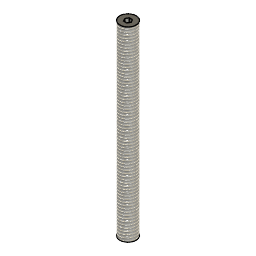
DoubleBarrelHotend (Autodesk Fusion 360 archive; units mm, degrees)
design "meltzone adapter"
Autodesk Fusion 360 part; units mm, degrees
sketch "Sketch1" plane through (0, 0, 0) normal (0, 0, 1) x (1, 0, 0)
  circle A0 centre (0, 0) radius 3
  circle A1 centre (0, 0) radius 1
  dimension "d1" = 6
  dimension "d2" = 2
  constraint coincident A0.centre A1.centre
  measures "d1" diameter of A0
  measures "d2" diameter of A1
extrude "Extrude1" add sketch "Sketch1" along normal blind 67
thread "Thread1" "ISO Metric profile 6.0 M6x1 M6x1 6g" major diameter 5.884 minor diameter 4.7435 pitch 1 angle 60 resizes the face on face at (2.9963, -0.1495, 44.6667)
sketch "Sketch2" plane through (0, 0, 67) normal (0, 0, 1) x (-1, 0, 0)
  circle A0 centre (0, 0) radius 1
  circle A1 centre (0, 0) radius 2.942
  line L0 (0.5774, -1) -> (1.1547, 0)
  line L1 (1.1547, 0) -> (0.5774, 1)
  line L2 (0.5774, 1) -> (-0.5774, 1)
  line L3 (-0.5774, 1) -> (-1.1547, 0)
  line L4 (-1.1547, 0) -> (-0.5774, -1)
  line L5 (-0.5774, -1) -> (0.5774, -1)
  constraint coincident A0.centre A1.centre
extrude "Extrude2" cut sketch "Sketch2" against normal blind 2 contours A0 | A0 L0 L1 | A0 L1 L2 | A0 L0 L5 | A0 L2 L3 | A0 L4 L5 | A0 L3 L4

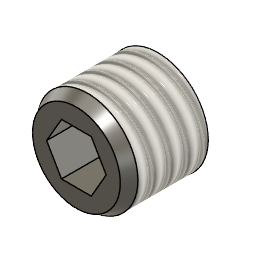
design "Hexagon Socket Set Screw ISO 4027 - M3 x 3 Steel 4.6 Plain"
description: Hexagon Socket Set Screw ISO 4027 - M3 x 3
part number: ISO 4027 - M3 x 3 Steel 4.6 Plain
Autodesk Fusion 360 part; units mm, degrees
sketch "Sketch1" plane through (0, 0, 0) normal (0, 1, 0) x (1, 0, 0)
  line L0 (-1.5, 0) -> (-1.5, 3)
  line L1 (0, 3) -> (0, 0)
  line L2 (0, 3) -> (-1.5, 3)
  line L3 (-1.5, 0) -> (0, 0)
  dimension "d107" = 3
  dimension "d136" = 3
  constraint vertical L0
  constraint perpendicular L0 L3
  constraint coincident L1.end L3
  constraint coincident L1.end L3.end
  constraint vertical L1
  constraint coincident L3.end L1
  measures "d107" distance of L2 L3
revolve "Revolve1" add sketch "Sketch1" angle 360 about axis through (0, 0, -3) along (0, 0, 1)
sketch "Sketch7" plane through (0, 0, 0) normal (0, 0, 1) x (1, 0, 0)
  line L0 (-0.866, 0) -> (-0.433, -0.75)
  line L1 (-0.433, -0.75) -> (0.433, -0.75)
  line L2 (0.433, -0.75) -> (0.866, 0)
  line L3 (0.866, 0) -> (0.433, 0.75)
  line L4 (0.433, 0.75) -> (-0.433, 0.75)
  line L5 (-0.433, 0.75) -> (-0.866, 0)
  dimension "d149" = 1.5
  constraint horizontal L2.end origin
  measures "d149" distance of L2 L5
extrude "Extrude4" cut sketch "Sketch7" against normal blind 1.2
extrude "Extrude5" cut 1 faces at (0.1443, -0.25, -1.2) along direction (0, 0, -1) blind 1.2 draft -60
thread "Thread2" "ISO Metric profile 3.0 M3x0.5 M3x0.5 6g" major diameter 2.927 minor diameter 2.3555 pitch 0.5 angle 60 resizes the face on face at (-1.4925, 0.1494, -2)
sketch "Sketch8" plane through (0, 0, 0) normal (0, 1, 0) x (1, 0, 0)
  line L0 (-1.53, 3) -> (-1.53, 2.3332)
  line L1 (-1.53, 2.3332) -> (-0.375, 3)
  line L2 (0, 3) -> (0, 0)
  line L3 (-1.53, 3) -> (0, 3)
  line L4 (0, 0) -> (-1.53, 0)
  line L5 (-1.53, 0) -> (-1.53, 0.4391)
  line L6 (-1.53, 0.4391) -> (-1.2765, 0)
  dimension "d130" = 60
  dimension "d138" = 60
  dimension "d145" = 0.375
  dimension "d146" = 1.53
  dimension "d147" = 0.2535
  dimension "d148" = 1.53
  constraint perpendicular L0 L3
  constraint coincident L2.start L3.end
  constraint horizontal L3
  constraint coincident L1.end L3
  constraint coincident L2.end L4.start
  constraint perpendicular L2 L4
  constraint perpendicular L4 L5
  constraint coincident L4 L6.end
  measures "d130" angle of L0 L1
  measures "d138" angle of L4 L6
  measures "d145" distance of L1.end L2
  measures "d146" distance of L0 L2.start
  measures "d147" distance of L5 L6.end
  measures "d148" distance of L2.end L5
revolve "Revolve4" cut sketch "Sketch8" angle 360 about axis through (0, 0, 1.75) along (0, 0, 1)
equation "adsk_nomlen = 3.00 mm"
equation "adsk_nomdia = 3.00 mm"
equation "adsk_phildepth = 1.20 mm"
equation "d102 = -adsk_phildepth"
equation "d107 = adsk_nomlen"
equation "adsk_endpointdia = 0.75 mm"
equation "adsk_startang = 60.00 deg"
equation "adsk_philwidth = 1.50 mm"
equation "d124 = -adsk_phildepth"
equation "d130 = adsk_startang"
equation "d136 = adsk_nomdia"
equation "adsk_chamang = 60.00 deg"
equation "d138 = adsk_chamang"
equation "d145 = adsk_endpointdia / 2"
equation "d146 = adsk_nomdia * 0.51"
equation "d147 = ( adsk_nomdia - adsk_philwidth * 1.155 ) / 5"
equation "d148 = adsk_nomdia * 0.51"
equation "d149 = adsk_philwidth"

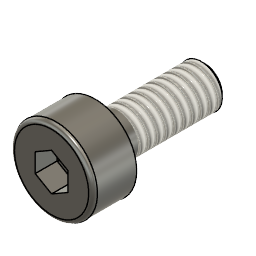
design "Hexagon Socket Head Cap Screw ISO 4762 - M2 x 5 Steel 4.6 Plain"
description: Hexagon Socket Head Cap Screw ISO 4762 - M2 x 5
part number: ISO 4762 - M2 x 5 Steel 4.6 Plain
Autodesk Fusion 360 part; units mm, degrees
sketch "Sketch1" plane through (0, 0, 0) normal (0, 1, 0) x (1, 0, 0)
  line L0 (-1, 0) -> (-1, 5)
  line L1 (-1, 5) -> (0, 5)
  line L2 (0, 5) -> (0, -2)
  line L3 (-1, 0) -> (-1.9, 0)
  line L4 (-1.9, 0) -> (-1.9, -2)
  line L5 (-1.9, -2) -> (0, -2)
  dimension "d9" = 2
  dimension "d106" = 2
  dimension "d107" = 5
  dimension "d116" = 3.8
  constraint perpendicular L0 L1
  constraint collinear origin L1.end L2.end
  constraint perpendicular L0 L3
  constraint coincident origin L3
  constraint vertical L2
  constraint coincident L2 L5.end
  constraint perpendicular L2 L5
  measures "d106" distance of L3 L5
  measures "d107" distance of origin L1
revolve "Revolve1" add sketch "Sketch1" angle 360 about axis through (0, 0, -5) along (0, 0, 1)
ref_plane "WorkPlane1" through (0, 0, 2) normal (0, 0, 1) x (1, 0, 0)
sketch "Sketch6" plane through (0, 0, 2) normal (0, 0, 1) x (1, 0, 0)
  line L0 (-0.75, 0.433) -> (-0.75, -0.433)
  line L1 (-0.75, -0.433) -> (0, -0.866)
  line L2 (0, -0.866) -> (0.75, -0.433)
  line L3 (0.75, -0.433) -> (0.75, 0.433)
  line L4 (0.75, 0.433) -> (0, 0.866)
  line L5 (0, 0.866) -> (-0.75, 0.433)
  dimension "d117" = 1.5
  constraint vertical L0
  measures "d117" distance of L0 L3
extrude "Extrude1" cut sketch "Sketch6" against normal blind 1
extrude "Extrude2" cut 1 faces at (0, -0.2887, 1) along direction (0, 0, -1) blind 1 draft -85
fillet "Fillet4" radius 0.2 1 edges at (-1.7714, 0.6871, 2)
thread "Thread3" "ISO Metric profile 2.0 M2x0.4 M2x0.4 6g" major diameter 1.9335 minor diameter 1.478 pitch 0.4 angle 60 resizes the face on face at (-0.9988, 0.0498, -3.3333) from (0, 0, -1) to (0, 0, -5)
sketch "Sketch7" plane through (0, 0, 0) normal (0, 1, 0) x (1, 0, 0)
  line L0 (-1.02, 5) -> (-1.02, 4.8)
  line L1 (-1.02, 4.8) -> (-0.82, 5)
  line L2 (0, 5) -> (0, -2)
  line L3 (-1.02, 5) -> (0, 5)
  dimension "d101" = 45
  dimension "d112" = 0.2
  dimension "d113" = 1.02
  constraint coincident L2.start L3.end
  constraint perpendicular L2 L3
  constraint coincident L1.end L3
  constraint perpendicular L0 L3
  measures "d101" angle of L0 L1
  measures "d112" distance of L0.end L3
  measures "d113" distance of L0 L2.start
revolve "Revolve3" cut sketch "Sketch7" angle 360 about axis through (0, 0, 1.75) along (0, 0, 1)
equation "d9 = adsk_nomdia"
equation "adsk_nomlen = 5.00 mm"
equation "adsk_headh = 2.00 mm"
equation "adsk_headdia = 3.80 mm"
equation "adsk_nomdia = 2.00 mm"
equation "adsk_philwidth = 1.50 mm"
equation "d31 = -adsk_phildepth"
equation "adsk_phildepth = 1.00 mm"
equation "d71 = adsk_headh"
equation "d76 = -adsk_phildepth"
equation "adsk_thrlen = 4.00 mm"
equation "d86 = adsk_nomdia * 0.1"
equation "adsk_startang = 45.00 deg"
equation "d101 = adsk_startang"
equation "adsk_pitch1 = 0.40 mm"
equation "adsk_startlen = 0.20 mm"
equation "d106 = adsk_headh"
equation "d107 = adsk_nomlen"
equation "d112 = adsk_startlen"
equation "d113 = adsk_nomdia * 0.51"
equation "d115 = min(adsk_thrlen; adsk_nomlen - 0.001 mm)"
equation "d116 = adsk_headdia"
equation "d117 = adsk_philwidth"
